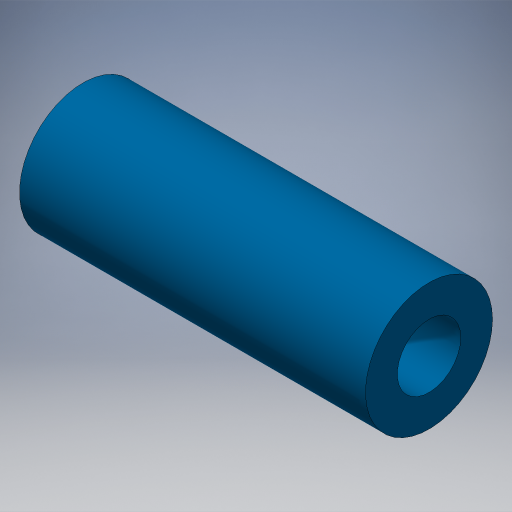
# Autodesk Inventor part: Rolle
Saved by Autodesk Inventor 2023.2 (Build 272271000, 271)
## iProperties
Company: CIDEON Software & Service GmbH & Co. KG
Created: 2022-11-29
Part Number: Rolle
Material: Polylactide (schwarz)
Document SubType Name: Modeling
Designer: A.Hess
Mass: 146.904 g
Surface Area: 224.31 cm^2
Volume: 102.73 cm^3
Density: 1.43 g/cm^3
Appearance: Generisch
CDN_Status: In Bearbeitung
Bauteiltyp: Fertigung
Gewicht: 0.00
Abmessungen: 0 x 0 x 0 mm
NORM: YES
CDN_KALK_STAERKE: 0,000
G_L: 0,000
G_W: 0,000
Fläche: 0.00
Author: A.Hess
Revision Number: 00
Autodesk Inventor part; units mm, degrees
ref_plane "YZ Plane" through (0, 0, 0) normal (1, 0, 0) x (0, 1, 0)
ref_plane "XZ Plane" through (0, 0, 0) normal (0, 1, 0) x (-1, 0, 0)
ref_plane "XY Plane" through (0, 0, 0) normal (0, 0, 1) x (1, 0, 0)
sketch "SK_Durchmesser" plane through (0, 0, 0) normal (1, 0, 0) x (0, 1, 0)
  circle A0 centre (0, 0) radius 10
  circle A1 centre (0, 0) radius 20
  dimension "d2" = 20
  dimension "d4" = 40
  constraints: 2 centre point, 2 coincident
  measures "d2" diameter of A0
  measures "d4" diameter of A1
extrude "Extrusion2" add sketch "SK_Durchmesser" along normal mid plane 109
equation "\"d2\" = Innendurchmesser"
equation "\"d4\" = Außendurchmesser"
equation "\"Außendurchmesser\" = 40"
equation "\"Innendurchmesser\" = 20"
